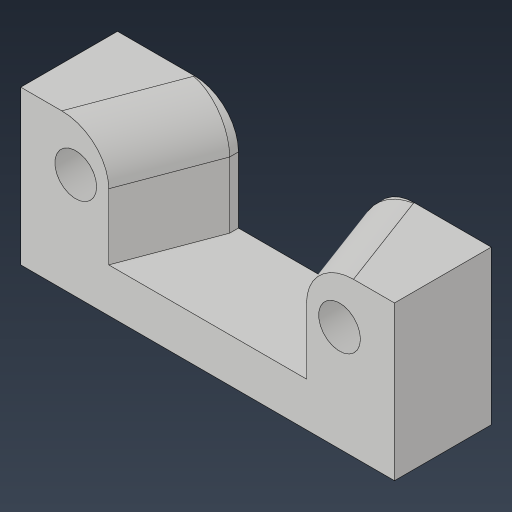
# Autodesk Inventor part: LED Schirm
Saved by Autodesk Inventor 2023.1 (Build 271208000, 208)
## iProperties
Part Number: LED Schirm
Material: Generisch
Document SubType Name: Modeling
Designer: rYan
Density: 1 g/cm^3
Appearance: Vorgabe
Mass: 0.323356 g
Surface Area: 5.34759 cm^2
Volume: 0.323356 cm^3
Author: rYan
Autodesk Inventor part; units mm, degrees
ref_plane "YZ Plane" through (0, 0, 0) normal (1, 0, 0) x (0, 1, 0)
ref_plane "XZ Plane" through (0, 0, 0) normal (0, 1, 0) x (-1, 0, 0)
ref_plane "XY Plane" through (0, 0, 0) normal (0, 0, 1) x (1, 0, 0)
sketch "Skizze1" plane through (0, 0, 0) normal (0, 1, 0) x (-1, 0, 0)
  line L0 (8.5, -4) -> (-8.5, -4)
  line L1 (-8.5, -4) -> (-8.5, 3)
  line L2 (-8.5, 3) -> (8.5, 3)
  line L3 (8.5, 3) -> (8.5, -4)
  line L4 (-11.9, 0) -> (11.9, 0) construction
  line L5 (0, -5.4) -> (0, 4.4) construction
  point P0 (0, 0)
  dimension "d0" = 17
  dimension "d1" = 7
  dimension "d60" = 3
  constraints: 8 end point, 2 parallel, 1 horizontal, 1 perpendicular, 1 other
  measures "d0" distance of L0.start L0.end
  measures "d1" distance of L0.end L1.end
  measures "d60" distance between parallel lines of L2 L4
extrude "Extrusion1" add sketch "Skizze1" along normal blind 4.4
sketch "Skizze2" plane through (0, 0, 0) normal (0, -1, 0) x (1, 0, 0)
  line L0 (-11.9, 0) -> (11.9, 0) projected
  line L1 (0, 4.4) -> (0, -5.4) projected
  point P0 (0, 0)
  point P1 (-6, 0.8)
  point P2 (6, 0.8)
  dimension "d5" = 0.8
  dimension "d6" = 6
  constraints: 1 symmetric about line
  measures "d5" distance from line of point (6, 0.8) L0
  measures "d6" distance from line of L1 point (6, 0.8)
hole "Bohrung1" at (-6, 0, 0.8) at (6, 0, 0.8) direction (0, 1, 0) diameter 1.9 end through all
sketch "Skizze5" plane through (0, 0, 0) normal (0, -1, 0) x (1, 0, 0)
  line L0 (8.5, -4) -> (-8.5, -4) projected
  line L1 (8.5, 3) -> (8.5, -4) projected
  line L2 (-8.5, -4) -> (8.5, -4)
  line L3 (8.5, -4) -> (8.5, -3)
  line L4 (8.5, -3) -> (-8.5, -3)
  line L5 (-8.5, -3) -> (-8.5, -4)
  point P0 (0, 0)
  dimension "d29" = 1
  constraints: 8 end point, 2 parallel, 1 horizontal, 1 perpendicular, 1 point on line
  measures "d29" distance of L4.end L0.end
extrude "Extrusion4" [suppressed]
sketch "Skizze6" plane through (0, 0, 0) normal (0, -1, 0) x (1, 0, 0)
  line L0 (8.5, -4) -> (8.5, 3) projected
  line L1 (8.5, 3) -> (-8.5, 3) projected
  line L2 (-8.5, 3) -> (-8.5, -4) projected
  circle A0 centre (-6, 0.8) radius 0.95 projected
  circle A1 centre (6, 0.8) radius 0.95 projected
  line L3 (8.5, 3) -> (-8.5, 3) projected
  line L4 (-3, 3) -> (3, 3)
  line L5 (3, 3) -> (3, -2)
  line L6 (3, -2) -> (-3, -2)
  line L7 (-3, -2) -> (-3, 3)
  line L8 (0, 4.4) -> (0, -5.4) projected
  line L9 (-8.5, -4) -> (8.5, -4) projected
  point P0 (0, 0)
  point P1 (0, 3)
  dimension "d32" = 6
  dimension "d58" = 2
  dimension "d59" = 2
  constraints: 8 end point, 2 parallel, 1 horizontal, 1 perpendicular, 1 point on line, 1 other
  measures "d32" distance between parallel lines of L5 L7
  measures "d58" distance from line of point (0, 0) L6
  measures "d59" distance between parallel lines of L9 L6
extrude "Extrusion5" cut sketch "Skizze6" against normal through all contours L5 L6 L8 L1 | L6 L7 L1 L8
sketch "Skizze7" plane through (-8.5, -0.4, -2) normal (0, 0, 1) x (1, 0, 0)
  line L0 (0, 0) -> (1, 0)
  line L1 (1, 0) -> (1, 0.4)
  line L2 (1, 0.4) -> (0, 0.4)
  line L3 (0, 0.4) -> (0, 0)
  line L4 (17, 0) -> (0, 0) projected
  line L5 (11.5, 0.4) -> (17, 0.4) projected
  line L6 (17, 0) -> (16, 0)
  line L7 (16, 0) -> (16, 0.4)
  line L8 (16, 0.4) -> (17, 0.4)
  line L9 (17, 0.4) -> (17, 0)
  point P0 (8.5, 0.4)
  dimension "d35" = 1
  dimension "d36" = 1
  constraints: 16 end point, 4 parallel, 2 horizontal, 2 perpendicular, 1 collinear, 1 point on line
  measures "d35" distance of L1.end L2.end
  measures "d36" distance between parallel lines of L9 L7
extrude "Extrusion6" [suppressed]
chamfer "Fase4" [suppressed]
chamfer "Fase6" distance 1.5 distance2 4 1 edges at (-3, 0, 0.5) measured on face at (1, 0, -3.3333)
chamfer "Fase7" distance 1.5 distance2 4 1 edges at (3, 0, 0.5) measured on face at (1, 0, -3.3333)
fillet "Rundung3" radius 2 4 edges at (-3.75, 2, 3) (-3, 4.2, 3) (3.75, 2, 3) (3, 4.2, 3)
sketch "Skizze8" plane through (0, 0, 0) normal (0, -1, 0) x (1, 0, 0)
  line L0 (-3, 3) -> (-7.5, 3) projected
  line L1 (-7.5, 3) -> (-7.5, -2) projected
  line L2 (-7.5, -2) -> (-3, -2) projected
  line L3 (-3, -2) -> (-3, 3) projected
  circle A0 centre (-6, 1) radius 0.95 projected
  line L4 (3, 3) -> (3, -2) projected
  line L5 (3, -2) -> (7.5, -2) projected
  line L6 (7.5, -2) -> (7.5, 3) projected
  line L7 (7.5, 3) -> (3, 3) projected
  circle A1 centre (6, 1) radius 0.95 projected
  line L8 (-7.5, 3) -> (-7.5, -2) projected
  line L9 (-7.5, -2) -> (-3, -2) projected
  line L10 (-3, -2) -> (-3, 3) projected
  line L11 (-3, 3) -> (-7.5, 3) projected
  line L12 (7.5, -2) -> (7.5, 3) projected
  line L13 (3, 3) -> (3, -2) projected
  line L14 (3, -2) -> (7.5, -2) projected
  line L15 (7.5, 3) -> (3, 3) projected
equation "\"d5\" = d4"
equation "\"d4\" = 0.8"
